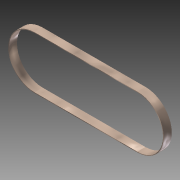
# Autodesk Inventor part: Rubber Band
Saved by Autodesk Inventor 2014 SP1 (Build 180222100, 222)
## iProperties
Created: 2014-11-19
Part Number: Rubber Band
Material: Generic
Document SubType Name: Modeling
Designer: AlecShufelt
Density: 1 g/cm^3
Appearance: Exterior - Beige
Author: AlecShufelt
Autodesk Inventor part; units mm, degrees
ref_plane "YZ Plane" through (0, 0, 0) normal (1, 0, 0) x (0, 1, 0)
ref_plane "XZ Plane" through (0, 0, 0) normal (0, 1, 0) x (-1, 0, 0)
ref_plane "XY Plane" through (0, 0, 0) normal (0, 0, 1) x (1, 0, 0)
sketch "Sketch1" plane through (0, 0, 0) normal (0, 0, 1) x (1, 0, 0)
  line L0 (0, 0) -> (57.15, 0)
  arc A0 (9.525, 9.525) -> (9.525, -9.525) centre (9.525, 0) ccw
  arc A1 (47.625, -9.525) -> (47.625, 9.525) centre (47.625, 0) ccw
  line L1 (11.7393, 9.525) -> (47.625, 9.525)
  line L2 (11.7393, -9.525) -> (47.625, -9.525)
  arc A2 (47.625, -9.779) -> (47.625, 9.779) centre (47.625, 0) ccw
  line L3 (9.525, 9.779) -> (47.625, 9.779)
  line L4 (9.525, -9.779) -> (47.625, -9.779)
  line L5 (11.7393, -9.525) -> (9.525, -9.525)
  line L6 (11.7393, 9.525) -> (9.525, 9.525)
  arc A3 (9.525, 9.779) -> (9.525, -9.779) centre (9.525, 0) ccw
  dimension "d0" = 57.15
  dimension "d2" = 19.558
  constraints: 14 end point, 10 point on circle, 6 tangent, 4 centre point, 2 coincident, 2 parallel, 2 point on line, 1 horizontal
  measures "d0" distance of L0.start L0.end
  measures "d2" diameter of A2
extrude "Extrusion1" add sketch "Sketch1" along normal blind 3
body "Solid1"
